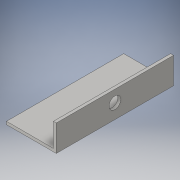
# Autodesk Inventor part: First Pivot Point
Saved by Autodesk Inventor 2016 (Build 200138000, 138)
## iProperties
Created: 2016-03-19
Part Number: First Pivot Point
Material: Generic
Document SubType Name: Modeling
Designer: matth_000
Density: 1 g/cm^3
Appearance: Default
Author: matth_000
Autodesk Inventor part; units mm, degrees
ref_plane "YZ Plane" through (0, 0, 0) normal (1, 0, 0) x (0, 1, 0)
ref_plane "XZ Plane" through (0, 0, 0) normal (0, 1, 0) x (-1, 0, 0)
ref_plane "XY Plane" through (0, 0, 0) normal (0, 0, 1) x (1, 0, 0)
sketch "Sketch1" plane through (0, 0, 0) normal (0, 1, 0) x (-1, 0, 0)
  line L0 (0, 0) -> (53.975, 0)
  line L1 (53.975, 0) -> (53.975, -127)
  line L2 (53.975, -127) -> (0, -127)
  line L3 (0, -127) -> (0, 0)
  dimension "d0" = 53.975
  dimension "d1" = 127
  constraints: 8 end point, 2 parallel, 1 horizontal, 1 perpendicular
  measures "d0" distance of L1.end L2.end
  measures "d1" distance of L0.end L1.end
extrude "Extrusion1" add sketch "Sketch1" along normal blind 3.175
sketch "Sketch2" plane through (0, 3.175, 0) normal (0, 1, 0) x (1, 0, 0)
  line L0 (0, 127) -> (-53.975, 127) projected
  line L1 (0, 0) -> (-3.175, 0)
  line L2 (-3.175, 0) -> (-3.175, 127)
  line L3 (-3.175, 127) -> (0, 127)
  line L4 (0, 127) -> (0, 0)
  dimension "d4" = 3.175
  constraints: 8 end point, 2 parallel, 1 horizontal, 1 perpendicular, 1 point on line
  measures "d4" distance of L2.end L3.end
extrude "Extrusion2" add sketch "Sketch2" along normal blind 25.4
sketch "Sketch3" plane through (-3.175, 3.175, -127) normal (-1, 0, 0) x (0, 0, 1)
  circle A0 centre (63.5, 12.7) radius 6.35
  line L0 (0, 25.4) -> (127, 25.4) projected
  line L1 (0, 0) -> (0, 25.4) projected
  point P0 (127, -3.175)
  dimension "d7" = 12.7
  dimension "d8" = 12.7
  dimension "d9" = 63.5
  constraints: 1 centre point
  measures "d7" diameter of A0
  measures "d8" distance from line of L0 A0.centre
  measures "d9" distance from line of L1 A0.centre
extrude "Extrusion3" cut sketch "Sketch3" against normal blind 3.175
body "Solid1"
